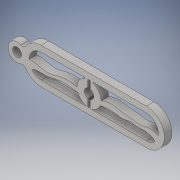
# Autodesk Inventor part: Key2
Saved by Autodesk Inventor 2016 (Build 200138000, 138)
## iProperties
Created: 2017-09-07
Part Number: Key2
Material: Generic
Document SubType Name: Modeling
Designer: Juan Alvarez
Density: 1 g/cm^3
Appearance: Default
Author: Juan Alvarez
Autodesk Inventor part; units mm, degrees
ref_plane "YZ Plane" through (0, 0, 0) normal (1, 0, 0) x (0, 1, 0)
ref_plane "XZ Plane" through (0, 0, 0) normal (0, 1, 0) x (-1, 0, 0)
ref_plane "XY Plane" through (0, 0, 0) normal (0, 0, 1) x (1, 0, 0)
sketch "Sketch1" plane through (0, 0, 0) normal (0, 0, 1) x (1, 0, 0)
  line L0 (-44.45, 0) -> (44.45, 0) construction
  line L1 (-44.45, -15.24) -> (44.45, -15.24)
  line L2 (44.45, 15.24) -> (-44.45, 15.24)
  arc A0 (44.45, -15.24) -> (44.45, 15.24) centre (44.45, 0) ccw
  circle A1 centre (-64.77, 0) radius 3.81
  arc A2 (-61.4643, 6.8656) -> (-61.4643, -6.8656) centre (-64.77, 0) ccw
  arc A3 (-44.45, 15.24) -> (-57.3909, 8.0493) centre (-44.45, 0) ccw
  arc A4 (-57.3909, -8.0493) -> (-44.45, -15.24) centre (-44.45, 0) ccw
  arc A5 (-61.4643, 6.8656) -> (-57.3909, 8.0493) centre (-60.0869, 9.7263) ccw
  arc A6 (-57.3909, -8.0493) -> (-61.4643, -6.8656) centre (-60.0869, -9.7263) ccw
  line L3 (-14.1826, 0) -> (-25.4036, 2.3152) construction
  line L4 (-25.4036, 2.3152) -> (-34.5348, -2.217) construction
  line L5 (-34.5348, -2.217) -> (-40.6596, -3.81) construction
  line L6 (-40.6596, -3.81) -> (-49.8132, 1.0589) construction
  line L7 (-49.8132, 1.0589) -> (-54.61, 0) construction
  spline S0 degree 4 poles (-14.1826, 0) (-25.4036, 2.3152) (-34.5348, -2.217) (-40.6596, -3.81) (-49.8132, 1.0589) (-54.61, 0) knots 1 1 1 1 1 2 3 3 3 3 3
  line L8 (-13.399, -3.9217) -> (-25.4036, -1.3756) construction
  line L9 (-25.4036, -1.3756) -> (-34.5348, -3.81) construction
  line L10 (-34.5348, -3.81) -> (-40.6596, -6.6774) construction
  line L11 (-40.6596, -6.6774) -> (-49.8132, -3.81) construction
  line L12 (-49.8132, -3.81) -> (-52.2116, -6.5561) construction
  spline S1 degree 4 poles (-13.399, -3.9217) (-25.4036, -1.3756) (-34.5348, -3.81) (-40.6596, -6.6774) (-49.8132, -3.81) (-52.2116, -6.5561) knots 1 1 1 1 1 2 3 3 3 3 3
  line L13 (6.2286, 0) -> (14.6914, 3.81) construction
  line L14 (14.6914, 3.81) -> (24.7367, -1.3756) construction
  line L15 (24.7367, -1.3756) -> (32.9178, 2.3152) construction
  line L16 (32.9178, 2.3152) -> (39.5623, -3.81) construction
  line L17 (39.5623, -3.81) -> (47.4662, 2.3152) construction
  line L18 (47.4662, 2.3152) -> (54.5164, -1.3756) construction
  spline S2 degree 4 poles (6.2286, 0) (14.6914, 3.81) (24.7367, -1.3756) (32.9178, 2.3152) (39.5623, -3.81) (47.4662, 2.3152) (54.5164, -1.3756) knots 1 1 1 1 1 2 3 4 4 4 4 4
  line L19 (5.445, -3.9217) -> (14.6691, -1.4873) construction
  line L20 (14.6691, -1.4873) -> (24.7144, -6.6711) construction
  line L21 (24.7144, -6.6711) -> (30.6822, 0) construction
  line L22 (30.6822, 0) -> (34.4324, -6.3846) construction
  line L23 (34.4324, -6.3846) -> (45.6585, -1.3756) construction
  line L24 (45.6585, -1.3756) -> (52.7088, -6.7823) construction
  line L25 (52.7088, -6.7823) -> (50.8485, -7.892) construction
  spline S3 degree 4 poles (5.445, -3.9217) (14.6691, -1.4873) (24.7144, -6.6711) (30.6822, 0) (34.4324, -6.3846) (45.6585, -1.3756) (52.7088, -6.7823) (50.8485, -7.892) knots 1 1 1 1 1 2 3 4 5 5 5 5 5
  line L26 (-3.0137, 10.16) -> (-3.0137, 3.8871)
  line L27 (-3.0137, -3.8871) -> (-3.0137, -10.16)
  line L28 (-4.9403, 10.16) -> (-4.9403, 3.8871)
  line L29 (-4.9403, -3.8871) -> (-4.9403, -10.16)
  line L30 (-44.45, 10.16) -> (-7.4149, 10.16)
  line L31 (-0.3615, 10.16) -> (44.45, 10.16)
  arc A7 (-4.9403, 3.8871) -> (-4.9403, -3.8871) centre (-3.977, 0) ccw
  arc A8 (-3.0137, -3.8871) -> (-3.0137, 3.8871) centre (-3.977, 0) ccw
  line L32 (44.45, -10.16) -> (-1.5866, -10.16)
  line L33 (-6.3674, -10.16) -> (-44.45, -10.16)
  arc A9 (-7.5378, 9.5642) -> (-14.1826, 0) centre (-3.977, 0) ccw
  arc A10 (-13.399, -3.9217) -> (-6.3674, -9.9217) centre (-3.977, 0) ccw
  arc A11 (-44.45, 10.16) -> (-54.61, 0) centre (-44.45, 0) ccw
  arc A12 (-52.2116, -6.5561) -> (-44.45, -10.16) centre (-44.45, 0) ccw
  arc A13 (-1.5866, -9.9217) -> (5.445, -3.9217) centre (-3.977, 0) ccw
  arc A14 (6.2286, 0) -> (-0.4796, 9.5876) centre (-3.977, 0) ccw
  arc A15 (44.45, -10.16) -> (51.1526, -7.6355) centre (44.45, 0) ccw
  arc A16 (54.5164, -1.3756) -> (44.45, 10.16) centre (44.45, 0) ccw
  line L34 (-6.3674, -9.9217) -> (-6.3674, -10.16)
  line L35 (-1.5866, -9.9217) -> (-1.5866, -10.16)
  line L36 (-7.4149, 10.16) -> (-7.5378, 9.5642)
  line L37 (-0.3615, 10.16) -> (-0.4796, 9.5876)
  line L38 (-4.9403, 10.16) -> (-3.0137, 10.16)
  line L39 (-4.9403, -10.16) -> (-3.0137, -10.16)
  point P0 (0, 0)
  point P1 (0, 0)
  dimension "d0" = 88.9
  dimension "d1" = 15.24
  dimension "d3" = 3.81
  dimension "d4" = 3.81
  dimension "d5" = 20.32
  dimension "d6" = 3.175
  dimension "d8" = 15.24
  constraints: 36 end point, 33 point on circle, 17 centre point, 8 tangent, 6 parallel, 3 horizontal, 3 point on line, 2 coincident, 1 equal radius, 1 horizontal alignment, 1 midpoint, 1 perpendicular, 1 vertical, 14 other
  measures "d0" distance of L0.start L0.end
  measures "d1" radius of A0
  measures "d3" radius of A1
  measures "d4" radial gap between concentric circles of A1 A2
  measures "d5" distance of L0.start A1.centre
  measures "d6" radius of A5
  measures "d8" radius of A3
extrude "Extrusion2" add sketch "Sketch1" along normal blind 6.35
body "Solid2"
